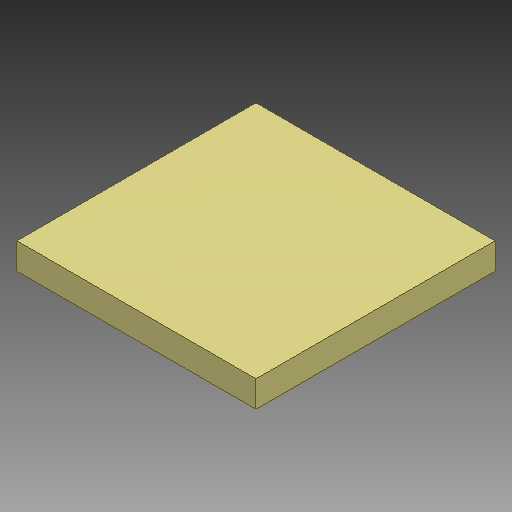
# Autodesk Inventor part: MEGA8-AI
Saved by Autodesk Inventor 2017.3 (Build 213256000, 256)
## iProperties
Part Number: MEGA8-AI
Material: Generisch
Document SubType Name: Modeling
Designer: Nils
Density: 1 g/cm^3
Appearance: TQFP32-08, MEGA8-AI
Author: Nils
Autodesk Inventor part; units mm, degrees
ref_plane "YZ Plane" through (0, 0, 0) normal (1, 0, 0) x (0, 1, 0)
ref_plane "XZ Plane" through (0, 0, 0) normal (0, 1, 0) x (-1, 0, 0)
ref_plane "XY Plane" through (0, 0, 0) normal (0, 0, 1) x (1, 0, 0)
sketch "TQFP32-08, MEGA8-AI_19" plane through (0, 0, 0) normal (0, 0, 1) x (1, 0, 0)
  line L0 (-4.5466, 4.5466) -> (4.5466, 4.5466)
  line L1 (4.5466, 4.5466) -> (4.5466, -4.5466)
  line L2 (4.5466, -4.5466) -> (-4.5466, -4.5466)
  line L3 (-4.5466, -4.5466) -> (-4.5466, 4.5466)
  constraints: 8 end point
extrude "Extrusion1" add sketch "TQFP32-08, MEGA8-AI_19" along normal blind 1
